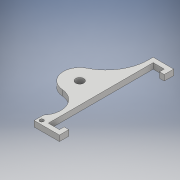
# Autodesk Inventor part: tab_clips
Saved by Autodesk Inventor 2018.3 (Build 223284000, 284)
## iProperties
Created: 2020-10-30
Part Number: tab_clips
Material: Generic
Document SubType Name: Modeling
Designer: chris
Density: 1 g/cm^3
Appearance: Default
Author: chris
Autodesk Inventor part; units mm, degrees
ref_plane "YZ Plane" through (0, 0, 0) normal (1, 0, 0) x (0, 1, 0)
ref_plane "XZ Plane" through (0, 0, 0) normal (0, 1, 0) x (-1, 0, 0)
sketch "Sketch1" plane through (0, 0, 0) normal (0, 0, 1) x (1, 0, 0)
  arc A0 (-7.692, 15.4959) -> (-1.3405, -17.248) centre (0, 0) ccw
  circle A1 centre (0, 0) radius 4.3
  line L0 (22.3, -55.7) -> (22.3, 55.7)
  line L1 (22.3, 55.7) -> (34.1, 55.7)
  line L2 (34.1, 60.7) -> (17.3, 60.7)
  line L3 (17.3, 60.7) -> (17.3, 55.7)
  line L4 (34.1, 60.7) -> (39.1, 60.7)
  line L5 (39.1, 60.7) -> (39.1, 50.7)
  line L6 (39.1, 50.7) -> (34.1, 50.7)
  line L7 (34.1, 50.7) -> (34.1, 55.7)
  line L8 (22.3, -55.7) -> (34.1, -55.7)
  line L9 (34.1, -60.7) -> (17.3, -60.7)
  line L10 (34.1, -60.7) -> (39.1, -60.7)
  line L11 (39.1, -60.7) -> (39.1, -50.7)
  line L12 (39.1, -50.7) -> (34.1, -50.7)
  line L13 (34.1, -50.7) -> (34.1, -55.7)
  arc A2 (-7.692, 15.4959) -> (17.3, 55.8032) centre (-27.7, 55.8032) ccw
  line L14 (22.3, -50.7) -> (22.3, -55.7)
  arc A3 (12.3, -50.7) -> (-1.3405, -17.248) centre (-2.9063, -37.3935) ccw
  circle A4 centre (16.3, -56.7) radius 2
  line L15 (12.3, -50.7) -> (12.3, -60.7)
  line L16 (12.3, -60.7) -> (17.3, -60.7)
  point P0 (17.3, -55.8032)
  constraints: 34 end point, 6 parallel, 6 point on circle, 5 centre point, 4 horizontal, 3 perpendicular, 2 tangent, 1 coincident, 1 point on line, 1 vertical, 1 other
extrude "Extrusion3" add sketch "Sketch1" along normal blind 6
ref_plane "Work Plane2" through (-17.3, 0, 0) normal (1, 0, 0) x (0, 1, 0)
sketch "Sketch3" plane through (-17.3, 0, 0) normal (1, 0, 0) x (0, 1, 0)
  circle A0 centre (0, 2.9763) radius 1.5
  point P0 (0, 0)
  constraints: 1 centre point
extrude "Extrusion4" cut sketch "Sketch3" along normal blind 8
body "Solid2"
